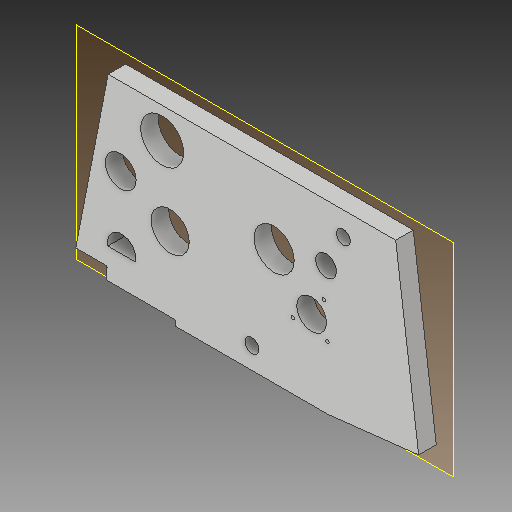
# Autodesk Inventor part: Part11.ipt-01
Saved by Autodesk Inventor 2018 (Build 220112000, 112)
## iProperties
Created: 2018-05-29
Part Number: Part11.ipt-01
Material: Generic
Document SubType Name: Modeling
Designer: p446024
Density: 1 g/cm^3
Appearance: Default
Author: p446024
Autodesk Inventor part; units mm, degrees
ref_plane "YZ Plane" through (0, 0, 0) normal (1, 0, 0) x (0, 1, 0)
ref_plane "XZ Plane" through (0, 0, 0) normal (0, 1, 0) x (-1, 0, 0)
ref_plane "XY Plane" through (0, 0, 0) normal (0, 0, 1) x (1, 0, 0)
ref_plane "Work Plane1" through (0, 0, 0) normal (0, 0, 1) x (1, 0, 0)
sketch "Sketch1" plane through (0, 0, 0) normal (0, 0, 1) x (1, 0, 0)
  circle A0 centre (64.078, -33.7875) radius 2.5 projected
  circle A1 centre (113.8201, -38.8599) radius 2.5 projected
  circle A2 centre (108.7476, 10.8821) radius 2.5 projected
  circle A3 centre (91.0159, -16.0557) radius 21.5 projected
  circle A4 centre (136.9222, 103.1056) radius 10 projected
  circle A5 centre (-113.0778, -14.3944) radius 27.5 projected
  circle A6 centre (-124.7161, 93.1056) radius 31 projected
  circle A7 centre (111.9222, 55.1056) radius 15 projected
  arc A8 (-163.0778, -77.8944) -> (-203.0778, -77.8944) centre (-183.0778, -73.3944) ccw projected
  line L0 (-203.0778, -77.8944) -> (-163.0778, -77.8944) projected
  circle A9 centre (4.8797, -98.3944) radius 10 projected
  circle A10 centre (36.9222, 38.038) radius 29 projected
  line L1 (-105.1203, -129.3944) -> (114.8797, -129.3944) projected
  line L2 (114.8797, -129.3944) -> (245.5334, -114.7214) projected
  line L3 (245.5334, -114.7214) -> (212.3797, 137.1056) projected
  line L4 (212.3797, 137.1056) -> (-202.6203, 137.1056) projected
  line L5 (-202.6203, 137.1056) -> (-249.3685, -103.3931) projected
  line L6 (-249.3685, -103.3931) -> (-206.3685, -103.3931) projected
  arc A11 (-204.3685, -105.3931) -> (-206.3685, -103.3931) centre (-206.3685, -105.3931) ccw projected
  line L7 (-204.3685, -105.3931) -> (-204.3685, -121.3931) projected
  line L8 (-204.3685, -121.3931) -> (-107.1203, -121.3931) projected
  arc A12 (-105.1203, -123.3931) -> (-107.1203, -121.3931) centre (-107.1203, -123.3931) ccw projected
  line L9 (-105.1203, -123.3931) -> (-105.1203, -129.3944) projected
  point P0 (0, 0)
extrude "Extrusion1" add sketch "Sketch1" along normal blind 25.4
sketch "Sketch2" plane through (0, 0, 25.4) normal (0, 0, 1) x (1, 0, 0)
  circle A0 centre (-184.4709, 24.8028) radius 22.2192
  point P0 (0, 0)
  dimension "Hole" = 44.4384
  constraints: 1 centre point
  measures "Hole" diameter of A0
extrude "Extrusion2" cut sketch "Sketch2" against normal through all
body "Solid1"
